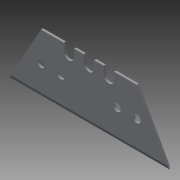
# Autodesk Inventor part: lametta
Saved by Autodesk Inventor 2014 SP2 (Build 180246200, 246)
## iProperties
Created: 2019-05-11
Part Number: lametta
Material: Generic
Document SubType Name: Modeling
Designer: GauchoHP
Density: 1 g/cm^3
Appearance: Default
Author: GauchoHP
Autodesk Inventor part; units mm, degrees
ref_plane "YZ Plane" through (0, 0, 0) normal (1, 0, 0) x (0, 1, 0)
ref_plane "XZ Plane" through (0, 0, 0) normal (0, 1, 0) x (-1, 0, 0)
ref_plane "XY Plane" through (0, 0, 0) normal (0, 0, 1) x (1, 0, 0)
sketch "Sketch1" plane through (0, 0, 0) normal (0, 1, 0) x (-1, 0, 0)
  line L0 (-20.518, 5.4955) -> (31.982, 5.4955)
  line L1 (31.982, 5.4955) -> (31.982, -13.5045)
  line L2 (31.982, -13.5045) -> (-20.518, -13.5045)
  line L3 (-20.518, -13.5045) -> (-20.518, 5.4955)
  line L4 (-10.018, 5.4955) -> (21.482, 5.4955)
  line L5 (21.482, -13.5045) -> (-10.018, -13.5045)
  line L6 (-20.518, -13.5045) -> (-10.018, 5.4955)
  line L7 (31.982, -13.5045) -> (21.482, 5.4955)
  line L8 (21.482, 5.4955) -> (13.982, 5.4955)
  line L9 (13.982, 5.4955) -> (13.982, 2.9955)
  line L10 (13.982, -2.0045) -> (21.482, -2.0045)
  line L11 (21.482, -2.0045) -> (21.482, 5.4955)
  line L12 (-10.018, 5.4955) -> (-2.518, 5.4955)
  line L13 (-2.518, 5.4955) -> (-2.518, 2.6913)
  line L14 (-2.518, -2.0045) -> (-10.018, -2.0045)
  line L15 (-10.018, -2.0045) -> (-10.018, 5.4955)
  line L16 (0.882, 5.4955) -> (0.882, 2.9955)
  line L17 (10.582, 5.4955) -> (10.582, -9.9414)
  line L18 (-0.818, 4.2892) -> (-0.818, 2.9955)
  line L19 (12.282, 4.2892) -> (12.282, 1.012)
  arc A0 (10.582, 2.9955) -> (13.982, 2.9955) centre (12.282, 2.9955) ccw
  line L20 (13.982, 2.9955) -> (18.4278, 2.9955)
  line L21 (4.032, 5.4955) -> (4.032, 2.6913)
  line L22 (7.432, 5.4955) -> (7.432, 2.9955)
  line L23 (5.732, 4.2892) -> (5.732, 2.9955)
  circle A1 centre (21.482, -4.1545) radius 1.25
  circle A2 centre (14.982, -4.1545) radius 1.25
  line L24 (21.482, -4.1545) -> (26.8149, -4.1545)
  circle A3 centre (-3.518, -4.1545) radius 1.25
  circle A4 centre (-10.018, -4.1545) radius 1.25
  line L25 (-10.018, -13.5045) -> (-10.018, -5.4045)
  line L26 (-10.018, -2.9045) -> (-10.018, 5.4955)
  line L27 (21.482, 5.4955) -> (21.482, -2.9045)
  line L28 (21.482, -5.4045) -> (21.482, -13.5045)
  line L29 (-5.1292, 2.9955) -> (-2.518, 2.9955)
  line L30 (1.4208, 2.9955) -> (4.032, 2.9955)
  arc A5 (-2.518, 2.9955) -> (0.882, 2.9955) centre (-0.818, 2.9955) ccw
  arc A6 (4.032, 2.9955) -> (7.432, 2.9955) centre (5.732, 2.9955) ccw
  line L31 (0.882, 5.4955) -> (4.032, 5.4955)
  line L32 (4.032, 2.9955) -> (4.032, 5.4955)
  line L33 (7.432, 5.4955) -> (7.432, 2.9955)
  line L34 (7.432, 5.4955) -> (10.582, 5.4955)
  line L35 (10.582, 5.4955) -> (10.582, 2.9955)
  line L36 (-2.518, 5.4955) -> (0.882, 5.4955)
  line L37 (0.882, 5.4955) -> (0.882, 2.9955)
  line L38 (0.882, 2.9955) -> (-2.518, 2.9955)
  line L39 (-2.518, 2.9955) -> (-2.518, 5.4955)
  line L40 (10.582, 5.4955) -> (13.982, 5.4955)
  line L41 (13.982, 5.4955) -> (13.982, 2.9955)
  line L42 (13.982, 2.9955) -> (10.582, 2.9955)
  line L43 (10.582, 2.9955) -> (10.582, 5.4955)
  line L44 (4.032, 5.4955) -> (7.432, 5.4955)
  line L45 (7.432, 5.4955) -> (7.432, 2.9955)
  line L46 (7.432, 2.9955) -> (4.032, 2.9955)
  line L47 (4.032, 2.9955) -> (4.032, 5.4955)
  point P0 (0, 0)
  point P1 (4.032, -2.0045)
  dimension "d0" = 52.5
  dimension "d1" = 19
  dimension "d2" = 31.5
  dimension "d3" = 19
  dimension "d6" = 7.5
  dimension "d7" = 7.5
  dimension "d9" = 7.5
  dimension "d10" = 7.5
  dimension "d11" = 3.4
  dimension "d12" = 3.4
  dimension "d14" = 1.7
  dimension "d15" = 1.7
  dimension "d16" = 7.5
  dimension "d17" = 3.4
  dimension "d18" = 1.7
  dimension "d19" = 3.15
  dimension "d21" = 3.15
  dimension "d22" = 2.5
  dimension "d23" = 2.5
  dimension "d24" = 6.5
  dimension "d25" = 9.65
  dimension "d26" = 9.35
  dimension "d28" = 5.3329
  dimension "d29" = 2.5
  dimension "d30" = 2.5
  dimension "d31" = 6.5
  dimension "d33" = 9.65
  dimension "d38" = 1.7
  dimension "d39" = 1.7
  dimension "d40" = 1.7
  constraints: 96 end point, 21 parallel, 13 perpendicular, 11 point on circle, 8 point on line, 7 centre point, 7 horizontal, 2 collinear, 2 tangent
  measures "d0" distance of L1.end L2.end
  measures "d1" distance of L0.end L1.end
  measures "d2" distance of L5.start L5.end
  measures "d3" distance of L4.end L5.start
  measures "d6" distance of L10.end L10.start
  measures "d7" distance of L10.start L8.end
  measures "d9" distance of L14.start L14.end
  measures "d10" distance of L12.end L14.start
  measures "d11" distance between parallel lines of L13 L16
  measures "d12" distance between parallel lines of L9 L17
  measures "d14" distance between parallel lines of L16 L18
  measures "d15" distance between parallel lines of L9 L19
  measures "d16" distance of L21.start point (4.032, -2.004)
  measures "d17" distance between parallel lines of L21 L22
  measures "d18" distance between parallel lines of L22 L23
  measures "d19" distance between parallel lines of L16 L21
  measures "d21" distance between parallel lines of L17 L22
  measures "d22" diameter of A1
  measures "d23" diameter of A2
  measures "d24" distance of L24.start A2.centre
  measures "d25" distance from line of L0 L24.start
  measures "d26" distance from line of L2 L24.start
  measures "d28" distance of L24.start L24.end
  measures "d29" diameter of A3
  measures "d30" diameter of A4
  measures "d31" distance of A3.centre A4.centre
  measures "d33" distance from line of L0 A4.centre
  measures "d38" radius of A0
  measures "d39" radius of A5
  measures "d40" radius of A6
extrude "Extrusion1" add sketch "Sketch1" along normal blind 0.7 contours L15 L26 A4 L25 L2 L6 | L0 L13 A5 L16 L21 A6 L22 L17 A0 L9 L11 L27 A1 L28 L2 L25 A4 L26 L15 | L28 A1 L24 L7 L2 | L24 A1 L27 L11 L7
chamfer "Chamfer1" distance 0.35 distance2 1 1 edges at (-5.732, 0, -13.5045) measured on face at (-5.732, 0.5, -13.5045)
chamfer "Chamfer2" distance 1 distance2 0.35 1 edges at (-5.732, 0.7, -13.5045) measured on face at (-5.732, 0.7, -13.0045)
body "Solid1"
